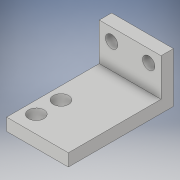
# Autodesk Inventor part: Abzugwinkel
Saved by Autodesk Inventor 2019 (Build 230136000, 136)
## iProperties
Created: 2021-03-08
Part Number: Abzugwinkel
Material: Generic
Document SubType Name: Modeling
Designer: Lukas
Density: 1 g/cm^3
Appearance: Default
Author: Lukas
Autodesk Inventor part; units mm, degrees
ref_plane "YZ Plane" through (0, 0, 0) normal (1, 0, 0) x (0, 1, 0)
ref_plane "XZ Plane" through (0, 0, 0) normal (0, 1, 0) x (-1, 0, 0)
ref_plane "XY Plane" through (0, 0, 0) normal (0, 0, 1) x (1, 0, 0)
sketch "Sketch1" plane through (0, 0, 0) normal (0, 0, 1) x (1, 0, 0)
  line L0 (-5, 4.05) -> (5, 4.05)
  line L1 (5, 4.05) -> (5, -4.05)
  line L2 (5, -4.05) -> (-5, -4.05)
  line L3 (-5, -4.05) -> (-5, 4.05)
  circle A0 centre (-3, 2.05) radius 1
  circle A1 centre (3, 2.05) radius 1
  point P0 (0, 0)
  point P1 (0, 4.05)
  point P2 (-5, 0)
  dimension "d0" = 10
  dimension "d1" = 8.1
  dimension "d2" = 6
  dimension "d3" = 2
  dimension "d4" = 2
  dimension "d5" = 2
  constraints: 8 end point, 2 centre point, 2 horizontal alignment, 2 midpoint, 2 parallel, 1 equal radius, 1 horizontal, 1 perpendicular, 1 vertical alignment
  measures "d0" distance of L0.start L0.end
  measures "d1" distance of L0.end L1.end
  measures "d2" distance of A1.centre A0.centre
  measures "d3" distance from line of L3 A0.centre
  measures "d4" diameter of A0
  measures "d5" distance from line of L0 A1.centre
extrude "Extrusion1" add sketch "Sketch1" along normal blind 2
sketch "Sketch2" plane through (0, 0, 2) normal (0, 0, 1) x (1, 0, 0)
  line L0 (5, -4.05) -> (5, 4.05) projected
  line L1 (-5, -4.05) -> (5, -4.05)
  line L2 (5, -4.05) -> (5, -2.05)
  line L3 (5, -2.05) -> (-5, -2.05)
  line L4 (-5, -2.05) -> (-5, -4.05)
  point P0 (0, 0)
  point P1 (4, 1)
  dimension "d8" = 2
  constraints: 8 end point, 2 parallel, 1 horizontal, 1 perpendicular, 2 other
  measures "d8" distance between parallel lines of L1 L3
extrude "Extrusion2" add sketch "Sketch2" along normal blind 15
sketch "Sketch3" plane through (-5, -2.05, 2) normal (0, 1, 0) x (1, 0, 0)
  circle A0 centre (2, -12.2) radius 1.25
  circle A1 centre (2, -8.2) radius 1.25
  line L0 (0, 0) -> (0, -15) projected
  line L1 (10, -15) -> (0, -15) projected
  line L2 (0, 0) -> (10, 0) projected
  point P0 (5, 2)
  dimension "d11" = 4
  dimension "d14" = 2.5
  dimension "d15" = 2
  dimension "d17" = 8.2
  constraints: 2 centre point, 1 equal radius, 1 vertical alignment
  measures "d11" distance of A1.centre A0.centre
  measures "d14" diameter of A1
  measures "d15" distance from line of L0 A1.centre
  measures "d17" distance from line of L2 A1.centre
extrude "Extrusion3" cut sketch "Sketch3" against normal through all
equation "\"d3\" = -0.5 * d2 + 0.5 * d0"
body "Solid1"
